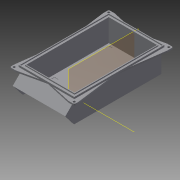
# Autodesk Inventor part: sensor3_1
Saved by Autodesk Inventor 2015 SP2 (Build 190223200, 223)
## iProperties
Created: 2016-02-11
Part Number: sensor3_1
Material: Generic
Document SubType Name: Modeling
Designer: mca20
Density: 1 g/cm^3
Appearance: Default
Author: mca20
Autodesk Inventor part; units mm, degrees
ref_plane "YZ Plane" through (0, 0, 0) normal (1, 0, 0) x (0, 1, 0)
ref_plane "XZ Plane" through (0, 0, 0) normal (0, 1, 0) x (-1, 0, 0)
ref_plane "XY Plane" through (0, 0, 0) normal (0, 0, 1) x (1, 0, 0)
sketch "Sketch1" plane through (0, 0, 0) normal (0, 1, 0) x (-1, 0, 0)
  line L0 (0, 0) -> (-63.34, 0)
  line L1 (-63.34, 0) -> (-63.34, -78.58)
  line L2 (-63.34, -78.58) -> (0, -78.58)
  line L3 (0, -78.58) -> (0, 0)
  line L4 (3, 3) -> (-66.34, 3)
  line L5 (-66.34, 3) -> (-66.34, -81.58)
  line L6 (-66.34, -81.58) -> (3, -81.58)
  line L7 (3, -81.58) -> (3, 3)
  dimension "d0" = 78.58
  dimension "d1" = 63.34
  dimension "d2" = 3
  constraints: 16 end point, 4 parallel, 2 perpendicular, 1 horizontal, 3 other
  measures "d0" distance between parallel lines of L2 L0
  measures "d1" distance between parallel lines of L1 L3
  measures "d2" distance between parallel lines of L3 L7
extrude "Extrusion1" add sketch "Sketch1" along normal blind 1.5 contours L3 L2 L1 L0 | L7 L6 L5 L4
sketch "Sketch2" plane through (0, 1.5, 0) normal (0, 1, 0) x (1, 0, 0)
  line L0 (-3, -3) -> (66.34, -3) projected
  line L1 (66.34, -3) -> (66.34, 81.58) projected
  line L2 (66.34, 81.58) -> (-3, 81.58) projected
  line L3 (-3, 81.58) -> (-3, -3) projected
  line L4 (0, 0) -> (63.34, 0)
  line L5 (63.34, 0) -> (63.34, 78.58)
  line L6 (63.34, 78.58) -> (0, 78.58)
  line L7 (0, 78.58) -> (0, 0)
  line L8 (0, 78.58) -> (5, 78.58)
  line L9 (5, 78.58) -> (5, 73.58)
  line L10 (5, 73.58) -> (0, 73.58)
  line L11 (0, 73.58) -> (0, 78.58)
  line L12 (63.34, 78.58) -> (58.34, 78.58)
  line L13 (58.34, 78.58) -> (58.34, 73.58)
  line L14 (58.34, 73.58) -> (63.34, 73.58)
  line L15 (63.34, 73.58) -> (63.34, 78.58)
  line L16 (0, 0) -> (5, 0)
  line L17 (5, 0) -> (5, 5)
  line L18 (5, 5) -> (0, 5)
  line L19 (0, 5) -> (0, 0)
  line L20 (63.34, 0) -> (58.34, 0)
  line L21 (58.34, 0) -> (58.34, 5)
  line L22 (58.34, 5) -> (63.34, 5)
  line L23 (63.34, 5) -> (63.34, 0)
  line L24 (-0.01, 73.57) -> (5.01, 73.57)
  line L25 (5.01, 73.57) -> (5.01, 78.59)
  line L26 (5.01, 78.59) -> (-0.01, 78.59)
  line L27 (-0.01, 78.59) -> (-0.01, 73.57)
  line L28 (63.35, 73.57) -> (58.33, 73.57)
  line L29 (58.33, 73.57) -> (58.33, 78.59)
  line L30 (58.33, 78.59) -> (63.35, 78.59)
  line L31 (63.35, 78.59) -> (63.35, 73.57)
  line L32 (63.35, 5.01) -> (58.33, 5.01)
  line L33 (58.33, 5.01) -> (58.33, -0.01)
  line L34 (58.33, -0.01) -> (63.35, -0.01)
  line L35 (63.35, -0.01) -> (63.35, 5.01)
  line L36 (-0.01, 5.01) -> (5.01, 5.01)
  line L37 (5.01, 5.01) -> (5.01, -0.01)
  line L38 (5.01, -0.01) -> (-0.01, -0.01)
  line L39 (-0.01, -0.01) -> (-0.01, 5.01)
  point P0 (0, 0)
  dimension "d5" = 3
  dimension "d6" = 5
  dimension "d7" = 5
  dimension "d8" = 5
  dimension "d9" = 5
  dimension "d10" = 5
  dimension "d11" = 5
  dimension "d12" = 5
  dimension "d13" = 5
  dimension "d16" = 0.01
  dimension "d19" = 0.01
  dimension "d20" = 0.01
  dimension "d21" = 0.01
  constraints: 72 end point, 16 parallel, 8 perpendicular, 4 horizontal, 15 other
  measures "d5" distance between parallel lines of L3 L7
  measures "d6" distance of L9.end L10.end
  measures "d7" distance of L8.end L9.end
  measures "d8" distance of L14.end L13.end
  measures "d9" distance of L13.end L12.end
  measures "d10" distance of L18.end L17.end
  measures "d11" distance of L17.end L16.end
  measures "d12" distance of L21.end L22.end
  measures "d13" distance of L20.end L21.end
  measures "d16" distance between parallel lines of L10 L24
  measures "d19" distance between parallel lines of L14 L28
  measures "d20" distance between parallel lines of L22 L32
  measures "d21" distance between parallel lines of L18 L36
extrude "Extrusion3" cut sketch "Sketch2" against normal blind 0.5 contours L7 L18 L17 L4 | L4 L37 L38 L39 L36 L7 | L17 L18 L7 L36 L37 L4 | L33 L32 L5 L22 L21 L4 | L4 L5 L32 L35 L34 L33 | L24 L27 L26 L25 L6 L7 | L7 L10 L9 L6 L25 L24 | L21 L22 L5 L4 | L7 L6 L9 L10 | L28 L29 L6 L13 L14 L5 | L5 L6 L29 L30 L31 L28 | L14 L13 L6 L5
sketch "Sketch3" plane through (0, 1.5, 0) normal (0, 1, 0) x (1, 0, 0)
  line L0 (-0.01, -0.01) -> (-0.01, 5.01) projected
  line L1 (-0.01, 5.01) -> (5.01, 5.01) projected
  line L2 (5.01, 5.01) -> (5.01, -0.01) projected
  line L3 (5.01, -0.01) -> (-0.01, -0.01) projected
  line L4 (63.35, 78.59) -> (63.35, 73.57) projected
  line L5 (63.35, 73.57) -> (58.33, 73.57) projected
  line L6 (58.33, 73.57) -> (58.33, 78.59) projected
  line L7 (58.33, 78.59) -> (63.35, 78.59) projected
  line L8 (5.01, 78.59) -> (5.01, 73.57) projected
  line L9 (5.01, 73.57) -> (-0.01, 73.57) projected
  line L10 (-0.01, 73.57) -> (-0.01, 78.59) projected
  line L11 (-0.01, 78.59) -> (5.01, 78.59) projected
  line L12 (58.33, -0.01) -> (58.33, 5.01) projected
  line L13 (58.33, 5.01) -> (63.35, 5.01) projected
  line L14 (63.35, 5.01) -> (63.35, -0.01) projected
  line L15 (63.35, -0.01) -> (58.33, -0.01) projected
  line L16 (-3, -3) -> (66.34, -3) projected
  line L17 (66.34, -3) -> (66.34, 81.58) projected
  line L18 (66.34, 81.58) -> (-3, 81.58) projected
  line L19 (-3, 81.58) -> (-3, -3) projected
  line L20 (-4, -4) -> (67.34, -4)
  line L21 (67.34, -4) -> (67.34, 82.58)
  line L22 (67.34, 82.58) -> (-4, 82.58)
  line L23 (-4, 82.58) -> (-4, -4)
  point P0 (0, 0)
  dimension "d22" = 1
  constraints: 8 end point, 3 other
  measures "d22" distance between parallel lines of L19 L23
extrude "Extrusion4" add sketch "Sketch3" along normal blind 30 and the other way blind 1.5 contours L23 L22 L21 L20
sketch "Sketch4" plane through (-4, 31.5, 4) normal (0, 0, 1) x (1, 0, 0)
  line L0 (1, 0) -> (70.34, 0)
  line L1 (70.34, 0) -> (70.34, -30)
  line L2 (70.34, -30) -> (1, -30)
  line L3 (1, -30) -> (1, 0)
  line L4 (71.34, -31.5) -> (0, -31.5) projected
  point P0 (4, -31.5)
  dimension "d27" = 1.5
  constraints: 8 end point, 2 parallel, 1 horizontal, 1 perpendicular
  measures "d27" distance between parallel lines of L4 L2
extrude "Extrusion5" cut sketch "Sketch4" against normal blind 1
ref_plane "Work Plane1" through (31.67, 0, -82.58) normal (1, 0, 0) x (0, 0, -1)
sketch "Sketch5" plane through (31.67, 0, -82.58) normal (1, 0, 0) x (0, 0, -1)
  point P0 (-82.58, 0)
ref_plane "Work Plane5" through (-4, 0, 4) normal (0, 0.7071068, -0.7071068) x (-1, 0, 0)
sketch "Sketch6" plane through (-4, 0, 4) normal (0, 0.7071068, -0.7071068) x (-1, 0, 0)
  line L0 (0, 0) -> (-71.34, 0)
  line L1 (-71.34, 0) -> (-71.34, 44.5517)
  line L2 (-71.34, 44.5517) -> (0, 44.5517)
  line L3 (0, 44.5517) -> (0, 0)
  point P0 (-4, -2.8284)
  constraints: 8 end point, 2 parallel, 1 horizontal, 1 perpendicular
extrude "Extrusion6" add sketch "Sketch6" along normal blind 1
sketch "Sketch7" plane through (67.34, 0, -82.58) normal (1, 0, 0) x (0, 0, -1)
  line L0 (-86.58, 1.4142) -> (-86.58, 31.5) projected
  line L1 (-86.58, 31.5) -> (-118.0828, 31.5028)
  line L2 (-118.0828, 31.5028) -> (-86.58, 0)
  line L3 (-118.0828, 31.5028) -> (-86.58, 0) projected
  line L4 (-86.58, 0) -> (-86.58, 31.5)
  point P0 (-82.58, 0)
  constraints: 6 end point, 2 collinear
extrude "Extrusion7" add sketch "Sketch7" against normal blind 1
mirror "Mirror1" about plane through (31.67, 0, -82.58) normal (1, 0, 0) of "Extrusion7"
sketch "Sketch8" plane through (66.34, 31.5027, 34.0885) normal (0, 1, -0.0000887) x (1, 0, 0)
  line L0 (-70.34, 0) -> (1, 0)
  line L1 (1, 0) -> (1, -1.4143)
  line L2 (1, -1.4143) -> (-70.34, -1.4143)
  line L3 (-70.34, -1.4143) -> (-70.34, 0)
  point P0 (-66.34, 34.0913)
  constraints: 8 end point, 2 parallel, 1 horizontal, 1 perpendicular
extrude "Extrusion8" cut sketch "Sketch8" along normal blind 1
sketch "Sketch9" plane through (0, 31.5, 0) normal (0, 1, 0) x (1, 0, 0)
  line L0 (-4, 82.58) -> (67.34, 82.58)
  line L1 (67.34, 82.58) -> (67.34, -35.5028)
  line L2 (67.34, -35.5028) -> (-4, -35.5028)
  line L3 (-4, -35.5028) -> (-4, 82.58)
  line L4 (-3, 81.58) -> (66.34, 81.58)
  line L5 (66.34, 81.58) -> (66.34, -34.0885)
  line L6 (66.34, -34.0885) -> (-3, -34.0885)
  line L7 (-3, -34.0885) -> (-3, 81.58)
  line L8 (68.34, 83.58) -> (-5, 83.58)
  line L9 (-5, 83.58) -> (-5, -36.5028)
  line L10 (-5, -36.5028) -> (68.34, -36.5028)
  line L11 (68.34, -36.5028) -> (68.34, 83.58)
  line L12 (-6, 84.58) -> (69.34, 84.58)
  line L13 (69.34, 84.58) -> (69.34, -37.5028)
  line L14 (69.34, -37.5028) -> (-6, -37.5028)
  line L15 (-6, -37.5028) -> (-6, 84.58)
  line L16 (65.34, 80.58) -> (-2, 80.58)
  line L17 (-2, 80.58) -> (-2, -33.0885)
  line L18 (-2, -33.0885) -> (65.34, -33.0885)
  line L19 (65.34, -33.0885) -> (65.34, 80.58)
  line L20 (-1, 79.58) -> (64.34, 79.58)
  line L21 (64.34, 79.58) -> (64.34, -32.0885)
  line L22 (64.34, -32.0885) -> (-1, -32.0885)
  line L23 (-1, -32.0885) -> (-1, 79.58)
  point P0 (0, 0)
  dimension "d39" = 1
  dimension "d40" = 1
  dimension "d41" = 1
  dimension "d42" = 1
  constraints: 48 end point, 12 parallel, 6 perpendicular, 2 horizontal, 12 other
  measures "d39" distance between parallel lines of L0 L8
  measures "d40" distance between parallel lines of L8 L12
  measures "d41" distance between parallel lines of L4 L16
  measures "d42" distance between parallel lines of L16 L20
extrude "Extrusion9" add sketch "Sketch9" along normal blind 1 contours L0 L1 L2 L3 | L4 L5 L6 L7 | L11 L10 L9 L8 | L12 L13 L14 L15 | L19 L18 L17 L16
sketch "Sketch10" plane through (0, 32.5, 0) normal (0, 1, 0) x (1, 0, 0)
  line L0 (64.34, 79.58) -> (64.34, -32.0885) projected
  line L1 (64.34, -32.0885) -> (-1, -32.0885) projected
  line L2 (-1, -32.0885) -> (-1, 79.58) projected
  line L3 (-1, 79.58) -> (64.34, 79.58) projected
  line L4 (69.34, 84.58) -> (-6, 84.58) projected
  line L5 (-6, 84.58) -> (-6, -37.5028) projected
  line L6 (-6, -37.5028) -> (69.34, -37.5028) projected
  line L7 (69.34, -37.5028) -> (69.34, 84.58) projected
  line L8 (-5, -36.5028) -> (-5, 83.58)
  line L9 (-5, 83.58) -> (68.34, 83.58)
  line L10 (68.34, 83.58) -> (68.34, -36.5028)
  line L11 (68.34, -36.5028) -> (-5, -36.5028)
  line L12 (-2, 80.58) -> (-2, -33.0885)
  line L13 (-2, -33.0885) -> (65.34, -33.0885)
  line L14 (65.34, -33.0885) -> (65.34, 80.58)
  line L15 (65.34, 80.58) -> (-2, 80.58)
  point P0 (0, 0)
  dimension "d45" = 1
  dimension "d46" = 1
  dimension "d108" = 111.6685
  constraints: 16 end point, 6 other
  measures "d45" distance between parallel lines of L5 L8
  measures "d46" distance between parallel lines of L2 L12
  measures "d108" distance between parallel lines of L1 L3
extrude "Extrusion10" add sketch "Sketch10" along normal blind 1.5
sketch "Sketch11" plane through (0, 31.5, 0) normal (0, -1, 0) x (1, 0, 0)
  line L0 (67.34, 35.5) -> (75.34, 35.5)
  line L1 (75.34, 35.5) -> (75.34, 43.5)
  line L2 (75.34, 43.5) -> (67.34, 43.5)
  line L3 (67.34, 43.5) -> (67.34, 35.5)
  line L4 (75.34, 43.5) -> (69.34, 43.5)
  line L5 (69.34, 43.5) -> (69.34, 37.5)
  line L6 (69.34, 37.5) -> (75.34, 37.5)
  line L7 (75.34, 37.5) -> (75.34, 43.5)
  line L8 (-4, -82.58) -> (67.34, -82.58) projected
  line L9 (67.34, 35.5) -> (-4, 35.5) projected
  line L10 (67.34, -82.58) -> (67.34, 35.5) projected
  line L11 (75.34, 37.5) -> (67.34, -23.54)
  line L12 (-4, -82.58) -> (-4, 35.5) projected
  line L13 (67.34, 43.5) -> (31.67, 35.5)
  line L14 (67.34, 35.5) -> (31.67, 35.5)
  line L15 (-3, 34.0858) -> (66.34, 34.0858) projected
  point P0 (0, 0)
  dimension "d49" = 8
  dimension "d50" = 8
  dimension "d51" = 6
  dimension "d52" = 6
  dimension "d53" = 118.08
  dimension "d54" = 59.04
  dimension "d55" = 71.34
  dimension "d56" = 35.67
  constraints: 22 end point, 5 parallel, 2 horizontal, 2 midpoint, 2 perpendicular
  measures "d49" distance of L2.end L1.end
  measures "d50" distance of L1.end L0.end
  measures "d51" distance of L6.end L5.end
  measures "d52" distance of L5.end L4.end
  measures "d53" distance between parallel lines of L8 L9
  measures "d54" distance from line of L11.end L9
  measures "d55" distance between parallel lines of L12 L10
  measures "d56" distance from line of L13.end L10
extrude "Extrusion11" add sketch "Sketch11" along normal blind 2 contours L3 L2 L5 L6 L11 L0 | L9 L13 L3 | L0 L11 L10 | L6 L5 L2 L1
sketch "Sketch13" plane through (67.34, 31.5, 35.5) normal (0, 0, -1) x (-1, 0, 0)
  line L0 (35.67, -2) -> (0, -2) projected
  line L1 (35.67, 0) -> (35.67, -2) projected
  line L2 (35.67, -0.0142) -> (0, -0.0142) projected
  line L3 (0, 0) -> (0, -2) projected
  point P0 (67.34, -31.5)
extrude "Extrusion12" add sketch "Sketch13" along normal blind 2
fillet "Fillet1" radius 2 1 edges at (75.34, 30.5, 43.5)
sketch "Sketch15" plane through (0, 31.5, 0) normal (0, 1, 0) x (1, 0, 0)
  line L0 (73.34, -43.5) -> (67.34, -43.5) projected
  arc A0 (73.34, -43.5) -> (75.34, -41.5) centre (73.34, -41.5) ccw projected
  line L1 (75.34, -37.5) -> (75.34, -41.5) projected
  line L2 (69.34, 8.28) -> (75.34, -37.5) projected
  line L3 (69.34, 8.28) -> (69.34, -37.5028) projected
  line L4 (69.34, -37.5028) -> (40.6, -37.5028) projected
  line L5 (67.34, -43.5) -> (40.6, -37.5028) projected
  line L6 (73.34, -43.5) -> (67.34, -43.5) projected
  line L7 (69.34, -37.5028) -> (75.34, -37.5028)
  line L8 (75.34, -37.5028) -> (75.34, -43.5028)
  line L9 (75.34, -43.5028) -> (69.34, -43.5028)
  line L10 (69.34, -43.5028) -> (69.34, -37.5028)
  circle A1 centre (72.34, -40.5028) radius 1.5
  point P0 (0, 0)
  dimension "d64" = 6
  dimension "d65" = 3
  constraints: 8 end point, 2 parallel, 1 centre point, 1 coincident, 1 horizontal, 1 perpendicular
  measures "d64" distance of L7.end L8.end
  measures "d65" diameter of A1
hole "Hole1" at (72.34, 31.5, 40.5028) direction (0, -1, 0) diameter 3 end through all
mirror "Mirror2" about plane through (31.67, 0, -82.58) normal (1, 0, 0) of "Extrusion11", "Extrusion12", "Fillet1"
sketch "Sketch14" plane through (67.34, 0, 4) normal (1, 0, 0) x (0, 0, -1)
  line L0 (-31.5, 31.5) -> (-31.5, 0)
  line L1 (-31.5, 0) -> (0, 0)
  line L2 (0, 0) -> (-31.5, 31.5)
  point P0 (4, 0)
  constraints: 6 end point, 1 perpendicular, 1 vertical
extrude "Extrusion13" add sketch "Sketch14" against normal blind 2
sketch "Sketch16" plane through (-4, 0, 4) normal (0, -0.7071068, 0.7071068) x (1, 0, 0)
  line L0 (71.34, 1.3859) -> (71.34, 41.7193) projected
  line L1 (0, 41.7193) -> (71.34, 41.7193)
  line L2 (71.34, 41.7193) -> (71.34, 39.7193)
  line L3 (71.34, 39.7193) -> (0, 39.7193)
  line L4 (0, 39.7193) -> (0, 41.7193)
  point P0 (4, -2.8284)
  dimension "d73" = 2
  constraints: 8 end point, 2 parallel, 1 horizontal, 1 perpendicular, 1 point on line
  measures "d73" distance of L1.end L2.end
extrude "Extrusion14" add sketch "Sketch16" along normal blind 20
sketch "Sketch17" plane through (67.34, 0, -82.58) normal (1, 0, 0) x (0, 0, -1)
  line L0 (-128.8079, 13.9437) -> (-118.08, 0)
  line L1 (-118.08, 0) -> (-118.08, 24.6716)
  line L2 (-118.08, 0) -> (-118.08, 24.6716) projected
  line L3 (-118.08, 24.6716) -> (-128.8079, 13.9437)
  line L4 (-118.08, 24.6716) -> (-114.6658, 28.0858) projected
  point P0 (-82.58, 0)
  constraints: 6 end point, 2 collinear
extrude "Extrusion15" add sketch "Sketch17" against normal blind 2
mirror "Mirror3" about plane through (31.67, 0, -82.58) normal (1, 0, 0) of "Extrusion15", "Extrusion13"
sketch "Sketch18" plane through (0, 31.5, 0) normal (0, -1, 0) x (1, 0, 0)
  line L0 (-4, -82.58) -> (-12, -82.58)
  line L1 (-12, -82.58) -> (-12, -90.58)
  line L2 (-12, -90.58) -> (-4, -90.58)
  line L3 (-4, -90.58) -> (-4, -82.58)
  line L4 (-12, -90.58) -> (-6, -90.58)
  line L5 (-6, -90.58) -> (-6, -84.58)
  line L6 (-6, -84.58) -> (-12, -84.58)
  line L7 (-12, -84.58) -> (-12, -90.58)
  line L8 (67.34, -82.58) -> (-4, -82.58) projected
  line L9 (31.67, -82.58) -> (-4, -90.58)
  line L10 (-4, -23.54) -> (-12, -82.58)
  line L11 (-4, -82.58) -> (-4, -23.54)
  point P0 (0, 0)
  dimension "d80" = 8
  dimension "d81" = 8
  dimension "d82" = 6
  dimension "d83" = 6
  constraints: 22 end point, 4 parallel, 2 horizontal, 2 perpendicular, 1 midpoint, 1 vertical
  measures "d80" distance of L2.end L1.end
  measures "d81" distance of L1.end L0.end
  measures "d82" distance of L6.end L5.end
  measures "d83" distance of L5.end L4.end
extrude "Extrusion16" add sketch "Sketch18" along normal blind 2
fillet "Fillet3" radius 2 1 edges at (-12, 30.5, -90.58)
mirror "Mirror5" about plane through (31.67, 0, -82.58) normal (1, 0, 0) of "Extrusion16", "Fillet3"
mirror "Mirror6" about plane through (31.67, 0, -82.58) normal (1, 0, 0) of "Hole1"
sketch "Sketch19" plane through (67.34, 31.5, -90.58) normal (0, 1, 0) x (1, 0, 0)
  line L0 (2, -6) -> (8, -6)
  line L1 (8, -6) -> (8, 0)
  line L2 (8, 0) -> (2, 0)
  line L3 (2, 0) -> (2, -6)
  circle A0 centre (5, -3) radius 1.5
  point P0 (-67.34, -90.58)
  dimension "d87" = 6
  dimension "d88" = 6
  dimension "d89" = 3
  constraints: 8 end point, 2 parallel, 1 centre point, 1 horizontal, 1 perpendicular
  measures "d87" distance of L2.end L1.end
  measures "d88" distance of L1.end L0.end
  measures "d89" diameter of A0
hole "Hole2" at (72.34, 31.5, -87.58) direction (0, -1, 0) diameter 3 end through all
mirror "Mirror7" about plane through (31.67, 0, -82.58) normal (1, 0, 0) of "Hole2"
sketch "Sketch20" plane through (-4, 0, 4) normal (0, -0.7071068, 0.7071068) x (1, 0, 0)
  line L0 (0, 22.2739) -> (0, -61.2213) projected
  line L1 (71.34, -61.2213) -> (71.34, 22.2739) projected
  circle A0 centre (35.67, 20) radius 4.925
  line L2 (69.34, 0) -> (2, 0) projected
  point P0 (4, -2.8284)
  dimension "d97" = 71.34
  dimension "d98" = 9.85
  dimension "d99" = 35.67
  dimension "d107" = 20
  constraints: 1 centre point
  measures "d97" distance between parallel lines of L0 L1
  measures "d98" diameter of A0
  measures "d99" distance from line of A0.centre L0
  measures "d107" distance from line of L2 A0.centre
hole "Hole3" at (31.67, 14.1421, 18.1421) direction (0, 0.7071068, -0.7071068) diameter 9.85 end through all
equation "\"d54\" = 0.5 * d53"
equation "\"d99\" = 0.5 * d97"
body "Solid1"
